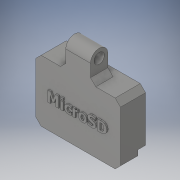
# Autodesk Inventor part: SDCardCover
Saved by Autodesk Inventor 2018 (Build 220112000, 112)
## iProperties
Created: 2019-01-13
Part Number: SDCardCover
Material: Generic
Document SubType Name: Modeling
Designer: tbrow
Density: 1 g/cm^3
Appearance: Default
Author: tbrow
## iProperties of the stored document SDCardCover_3DPrint.ipt
Created: 2019-01-15
Part Number: SDCardCover_3DPrint
Material: Generic
Document SubType Name: Modeling
Designer: tbrow
Density: 1 g/cm^3
Appearance: Default
Author: tbrow
Autodesk Inventor part; units mm, degrees
note: some values were not read from the file. Chosen so that the rebuilt part matches the saved one: direction of "Emboss1".
ref_plane "YZ Plane" through (0, 0, 0) normal (1, 0, 0) x (0, 1, 0)
ref_plane "XZ Plane" through (0, 0, 0) normal (0, 1, 0) x (-1, 0, 0)
ref_plane "XY Plane" through (0, 0, 0) normal (0, 0, 1) x (1, 0, 0)
sketch "Sketch1" plane through (0, 0, 0) normal (0, 0, 1) x (1, 0, 0)
  line L0 (0, 0) -> (0, 22.1234)
  line L1 (0, 22.1234) -> (10.795, 22.1234)
  line L2 (10.795, 22.1234) -> (10.795, 31.6484)
  line L3 (10.795, 31.6484) -> (19.685, 31.6484)
  line L4 (19.685, 31.6484) -> (19.685, 22.1234)
  line L5 (19.685, 22.1234) -> (30.48, 22.1234)
  line L6 (30.48, 22.1234) -> (30.48, 0)
  line L7 (30.48, 0) -> (0, 0)
  dimension "d0" = 10.795
  dimension "d1" = 9.525
  dimension "d2" = 8.89
  dimension "d3" = 10.795
  dimension "d17" = 31.6484
  constraints: 16 end point, 6 perpendicular, 2 point on line, 1 vertical
  measures "d0" distance of L4.end L5.end
  measures "d1" distance of L3.end L4.end
  measures "d2" distance of L2.end L3.end
  measures "d3" distance of L0.end L1.end
  measures "d17" distance between parallel lines of L7 L3
extrude "Extrusion1" add sketch "Sketch1" along normal blind 6.2484
sketch "Sketch2" plane through (19.685, 22.1234, 0) normal (1, 0, 0) x (0, 0, -1)
  circle A0 centre (-3.1242, 6.4008) radius 1.8542
  line L0 (0, 9.525) -> (-6.2484, 9.525) projected
  line L1 (-3.1242, 9.525) -> (-3.1242, 0) construction
  line L2 (0, 0) -> (-6.2484, 0) projected
  point P0 (0, -22.1234)
  dimension "d7" = 3.7084
  dimension "d8" = 3.1242
  constraints: 2 end point, 2 midpoint, 1 centre point, 1 point on line
  measures "d7" diameter of A0
  measures "d8" distance from line of L0 A0.centre
extrude "Extrusion2" cut sketch "Sketch2" against normal through all
fillet "Fillet1" radius 3.1242 2 edges at (15.24, 31.6484, 6.2484) (15.24, 31.6484, 0)
chamfer "Chamfer1" distance 1.905 angle 45 6 edges at (19.685, 22.1234, 3.1242) (10.795, 22.1234, 3.1242) (30.48, 22.1234, 3.1242) (0, 22.1234, 3.1242) (30.48, 0, 3.1242) (0, 0, 3.1242)
sketch "Sketch3" plane through (0, 0, 6.2484) normal (0, 0, 1) x (1, 0, 0)
  line L0 (4.3912, 13.1811) -> (26.0888, 13.1811) construction
  line L1 (26.0888, 13.1811) -> (26.0888, 8.9423) construction
  line L2 (26.0888, 8.9423) -> (4.3912, 8.9423) construction
  line L3 (4.3912, 8.9423) -> (4.3912, 13.1811) construction
  line L4 (4.3912, 11.0617) -> (26.0888, 11.0617) construction
  line L5 (15.24, 13.1811) -> (15.24, 8.9423) construction
  line L6 (19.685, 31.6484) -> (10.795, 31.6484) projected
  line L7 (15.24, 31.6484) -> (15.24, 0) construction
  line L8 (28.575, 0) -> (0, 0) projected
  line L9 (0, 0) -> (0, 20.2184) projected
  line L10 (0, 11.0617) -> (30.48, 11.0617) construction
  line L11 (30.48, 20.2184) -> (30.48, 1.905) projected
  line L12 (8.6766, 9.1982) -> (7.7257, 9.1982)
  line L13 (7.7257, 9.1982) -> (7.7257, 11.7238)
  line L14 (7.7257, 11.7238) -> (7.0341, 10.0936)
  line L15 (7.0341, 10.0936) -> (6.3795, 10.0936)
  line L16 (6.3795, 10.0936) -> (5.6879, 11.7238)
  line L17 (5.6879, 11.7238) -> (5.6879, 9.1982)
  line L18 (5.6879, 9.1982) -> (4.7864, 9.1982)
  line L19 (4.7864, 9.1982) -> (4.7864, 13.0082)
  line L20 (4.7864, 13.0082) -> (5.8886, 13.0082)
  line L21 (5.8886, 13.0082) -> (6.7346, 11.1279)
  line L22 (6.7346, 11.1279) -> (7.5744, 13.0082)
  line L23 (7.5744, 13.0082) -> (8.6766, 13.0082)
  line L24 (8.6766, 13.0082) -> (8.6766, 9.1982)
  line L25 (10.3099, 9.1982) -> (9.4146, 9.1982)
  line L26 (9.4146, 9.1982) -> (9.4146, 12.0727)
  line L27 (9.4146, 12.0727) -> (10.3099, 12.0727)
  line L28 (10.3099, 12.0727) -> (10.3099, 9.1982)
  line L29 (10.3377, 12.4833) -> (9.3899, 12.4833)
  line L30 (9.3899, 12.4833) -> (9.3899, 13.1811)
  line L31 (9.3899, 13.1811) -> (10.3377, 13.1811)
  line L32 (10.3377, 13.1811) -> (10.3377, 12.4833)
  spline S0 degree 2 poles (12.4033, 9.121) (12.0482, 9.121) (11.4585, 9.3001) (11.2393, 9.4853) knots 0 0 0 1 2 2 2
  spline S1 degree 2 poles (11.2393, 9.4853) (11.0262, 9.6737) (10.7854, 10.2387) (10.7854, 10.6216) knots 0 0 0 1 2 2 2
  spline S2 degree 2 poles (10.7854, 10.6216) (10.7854, 11.0353) (11.0448, 11.6126) (11.2702, 11.7979) knots 0 0 0 1 2 2 2
  spline S3 degree 2 poles (11.2702, 11.7979) (11.4832, 11.977) (12.0636, 12.1499) (12.3786, 12.1499) knots 0 0 0 1 2 2 2
  spline S4 degree 2 poles (12.3786, 12.1499) (12.6163, 12.1499) (13.0918, 12.0387) (13.3326, 11.9183) knots 0 0 0 1 2 2 2
  line L33 (13.3326, 11.9183) -> (13.3326, 11.1526)
  line L34 (13.3326, 11.1526) -> (13.2184, 11.1526)
  spline S5 degree 2 poles (13.2184, 11.1526) (13.1628, 11.2051) (13.0084, 11.3286) (12.9158, 11.378) knots 0 0 0 1 2 2 2
  spline S6 degree 2 poles (12.9158, 11.378) (12.817, 11.4336) (12.5731, 11.5077) (12.4218, 11.5077) knots 0 0 0 1 2 2 2
  spline S7 degree 2 poles (12.4218, 11.5077) (12.0791, 11.5077) (11.7024, 11.0291) (11.7024, 10.6216) knots 0 0 0 1 2 2 2
  spline S8 degree 2 poles (11.7024, 10.6216) (11.7024, 10.1893) (12.1038, 9.7632) (12.4372, 9.7632) knots 0 0 0 1 2 2 2
  spline S9 degree 2 poles (12.4372, 9.7632) (12.6071, 9.7632) (12.8602, 9.8404) (12.9529, 9.896) knots 0 0 0 1 2 2 2
  spline S10 degree 2 poles (12.9529, 9.896) (13.0424, 9.9485) (13.1721, 10.0658) (13.2184, 10.1121) knots 0 0 0 1 2 2 2
  line L35 (13.2184, 10.1121) -> (13.3326, 10.1121)
  line L36 (13.3326, 10.1121) -> (13.3326, 9.3433)
  spline S11 degree 2 poles (13.3326, 9.3433) (13.2554, 9.3094) (13.0547, 9.2229) (12.9498, 9.1951) knots 0 0 0 1 2 2 2
  spline S12 degree 2 poles (12.9498, 9.1951) (12.8201, 9.1581) (12.5916, 9.121) (12.4033, 9.121) knots 0 0 0 1 2 2 2
  line L37 (15.6884, 11.2236) -> (15.6143, 11.2236)
  spline S13 degree 2 poles (15.6143, 11.2236) (15.5618, 11.2421) (15.3673, 11.2607) (15.25, 11.2607) knots 0 0 0 1 2 2 2
  spline S14 degree 2 poles (15.25, 11.2607) (15.111, 11.2607) (14.7992, 11.1773) (14.6541, 11.1217) knots 0 0 0 1 2 2 2
  line L38 (14.6541, 11.1217) -> (14.6541, 9.1982)
  line L39 (14.6541, 9.1982) -> (13.7587, 9.1982)
  line L40 (13.7587, 9.1982) -> (13.7587, 12.0727)
  line L41 (13.7587, 12.0727) -> (14.6541, 12.0727)
  line L42 (14.6541, 12.0727) -> (14.6541, 11.659)
  spline S15 degree 2 poles (14.6541, 11.659) (14.7158, 11.7145) (14.932, 11.8874) (15.0215, 11.9399) knots 0 0 0 1 2 2 2
  spline S16 degree 2 poles (15.0215, 11.9399) (15.1203, 11.9986) (15.3796, 12.0819) (15.4939, 12.0819) knots 0 0 0 1 2 2 2
  spline S17 degree 2 poles (15.4939, 12.0819) (15.5371, 12.0819) (15.6452, 12.0758) (15.6884, 12.0727) knots 0 0 0 1 2 2 2
  line L43 (15.6884, 12.0727) -> (15.6884, 11.2236)
  spline S18 degree 2 poles (18.7883, 10.6339) (18.7883, 9.9238) (18.0133, 9.1087) (17.3063, 9.1087) knots 0 0 0 1 2 2 2
  spline S19 degree 2 poles (17.3063, 9.1087) (16.6023, 9.1087) (15.8212, 9.9238) (15.8212, 10.6339) knots 0 0 0 1 2 2 2
  spline S20 degree 2 poles (15.8212, 10.6339) (15.8212, 11.3502) (16.6023, 12.1622) (17.3063, 12.1622) knots 0 0 0 1 2 2 2
  spline S21 degree 2 poles (17.3063, 12.1622) (18.0102, 12.1622) (18.7883, 11.3471) (18.7883, 10.6339) knots 0 0 0 1 2 2 2
  spline S22 degree 2 poles (17.8713, 10.6277) (17.8713, 10.884) (17.7879, 11.2267) (17.7138, 11.3286) knots 0 0 0 1 2 2 2
  spline S23 degree 2 poles (17.7138, 11.3286) (17.6335, 11.4367) (17.4328, 11.52) (17.3063, 11.52) knots 0 0 0 1 2 2 2
  spline S24 degree 2 poles (17.3063, 11.52) (17.1828, 11.52) (16.9882, 11.4459) (16.908, 11.3409) knots 0 0 0 1 2 2 2
  spline S25 degree 2 poles (16.908, 11.3409) (16.8308, 11.2421) (16.7382, 10.8933) (16.7382, 10.6277) knots 0 0 0 1 2 2 2
  spline S26 degree 2 poles (16.7382, 10.6277) (16.7382, 10.3653) (16.8246, 10.0411) (16.8956, 9.9423) knots 0 0 0 1 2 2 2
  spline S27 degree 2 poles (16.8956, 9.9423) (16.9666, 9.8435) (17.1828, 9.7509) (17.3124, 9.7509) knots 0 0 0 1 2 2 2
  spline S28 degree 2 poles (17.3124, 9.7509) (17.4205, 9.7509) (17.6428, 9.8435) (17.7107, 9.9361) knots 0 0 0 1 2 2 2
  spline S29 degree 2 poles (17.7107, 9.9361) (17.7879, 10.0442) (17.8713, 10.356) (17.8713, 10.6277) knots 0 0 0 1 2 2 2
  spline S30 degree 2 poles (20.4926, 9.1303) (20.0542, 9.1303) (19.3934, 9.3001) (19.1094, 9.4236) knots 0 0 0 1 2 2 2
  line L44 (19.1094, 9.4236) -> (19.1094, 10.3313)
  line L45 (19.1094, 10.3313) -> (19.1958, 10.3313)
  spline S31 degree 2 poles (19.1958, 10.3313) (19.483, 10.0874) (20.1715, 9.825) (20.4957, 9.825) knots 0 0 0 1 2 2 2
  spline S32 degree 2 poles (20.4957, 9.825) (20.579, 9.825) (20.8476, 9.862) (20.9279, 9.8991) knots 0 0 0 1 2 2 2
  spline S33 degree 2 poles (20.9279, 9.8991) (21.0267, 9.9423) (21.1657, 10.0998) (21.1657, 10.2263) knots 0 0 0 1 2 2 2
  spline S34 degree 2 poles (21.1657, 10.2263) (21.1657, 10.3715) (20.9403, 10.5505) (20.7859, 10.5907) knots 0 0 0 1 2 2 2
  spline S35 degree 2 poles (20.7859, 10.5907) (20.5914, 10.6432) (20.1499, 10.7327) (19.9554, 10.8006) knots 0 0 0 1 2 2 2
  spline S36 degree 2 poles (19.9554, 10.8006) (19.5138, 10.955) (19.131, 11.483) (19.131, 11.8782) knots 0 0 0 1 2 2 2
  spline S37 degree 2 poles (19.131, 11.8782) (19.131, 12.4123) (20.0356, 13.0761) (20.7149, 13.0761) knots 0 0 0 1 2 2 2
  spline S38 degree 2 poles (20.7149, 13.0761) (21.0545, 13.0761) (21.7276, 12.9372) (21.9931, 12.8199) knots 0 0 0 1 2 2 2
  line L46 (21.9931, 12.8199) -> (21.9931, 11.9492)
  line L47 (21.9931, 11.9492) -> (21.9098, 11.9492)
  spline S39 degree 2 poles (21.9098, 11.9492) (21.6967, 12.1313) (21.0854, 12.3814) (20.7643, 12.3814) knots 0 0 0 1 2 2 2
  spline S40 degree 2 poles (20.7643, 12.3814) (20.6377, 12.3814) (20.4401, 12.3444) (20.3289, 12.295) knots 0 0 0 1 2 2 2
  spline S41 degree 2 poles (20.3289, 12.295) (20.2394, 12.2548) (20.1097, 12.0943) (20.1097, 11.9955) knots 0 0 0 1 2 2 2
  spline S42 degree 2 poles (20.1097, 11.9955) (20.1097, 11.8473) (20.3166, 11.6775) (20.613, 11.6096) knots 0 0 0 1 2 2 2
  spline S43 degree 2 poles (20.613, 11.6096) (20.8044, 11.5663) (21.1595, 11.483) (21.3633, 11.412) knots 0 0 0 1 2 2 2
  spline S44 degree 2 poles (21.3633, 11.412) (21.7585, 11.2668) (22.1444, 10.7852) (22.1444, 10.39) knots 0 0 0 1 2 2 2
  spline S45 degree 2 poles (22.1444, 10.39) (22.1444, 9.8219) (21.2521, 9.1303) (20.4926, 9.1303) knots 0 0 0 1 2 2 2
  spline S46 degree 2 poles (26.0347, 11.1001) (26.0347, 10.566) (25.5685, 9.7262) (25.2134, 9.5008) knots 0 0 0 1 2 2 2
  spline S47 degree 2 poles (25.2134, 9.5008) (24.917, 9.3094) (24.2192, 9.1982) (23.8271, 9.1982) knots 0 0 0 1 2 2 2
  line L48 (23.8271, 9.1982) -> (22.6353, 9.1982)
  line L49 (22.6353, 9.1982) -> (22.6353, 13.0082)
  line L50 (22.6353, 13.0082) -> (23.8148, 13.0082)
  spline S48 degree 2 poles (23.8148, 13.0082) (24.2161, 13.0082) (24.917, 12.9063) (25.2257, 12.7087) knots 0 0 0 1 2 2 2
  spline S49 degree 2 poles (25.2257, 12.7087) (25.5993, 12.4679) (26.0347, 11.6528) (26.0347, 11.1001) knots 0 0 0 1 2 2 2
  spline S50 degree 2 poles (25.0528, 11.1063) (25.0528, 11.483) (24.7935, 12.0202) (24.528, 12.1715) knots 0 0 0 1 2 2 2
  spline S51 degree 2 poles (24.528, 12.1715) (24.3335, 12.2765) (23.9074, 12.2981) (23.611, 12.2981) knots 0 0 0 1 2 2 2
  line L51 (23.611, 12.2981) -> (23.5925, 12.2981)
  line L52 (23.5925, 12.2981) -> (23.5925, 9.9114)
  line L53 (23.5925, 9.9114) -> (23.611, 9.9114)
  spline S52 degree 2 poles (23.611, 9.9114) (23.9321, 9.9114) (24.3736, 9.933) (24.5743, 10.0596) knots 0 0 0 1 2 2 2
  spline S53 degree 2 poles (24.5743, 10.0596) (24.8089, 10.2078) (25.0528, 10.7296) (25.0528, 11.1063) knots 0 0 0 1 2 2 2
  point P0 (30.48, 0)
  point P1 (0, 22.1234)
  point P2 (30.48, 22.1234)
  constraints: 8 end point, 6 midpoint, 2 collinear, 2 point on line, 2 other
emboss "Emboss1" sketch "Sketch3" operation add depth 0.508 direction (0, 0, -1)
sketch "Sketch4" plane through (0, 0, 0) normal (0, 0, -1) x (-1, 0, 0)
  line L0 (-21.59, 22.1234) -> (-8.89, 22.1234)
  line L1 (-1.905, 22.1234) -> (-8.89, 22.1234) projected
  line L2 (-1.905, 22.1234) -> (0, 20.2184) projected
  line L3 (0, 1.905) -> (0, 20.2184) projected
  line L4 (0, 1.905) -> (-1.905, 0) projected
  line L5 (-28.575, 0) -> (-1.905, 0) projected
  line L6 (-28.575, 0) -> (-30.48, 1.905) projected
  line L7 (-30.48, 20.2184) -> (-30.48, 1.905) projected
  line L8 (-30.48, 20.2184) -> (-28.575, 22.1234) projected
  line L9 (-21.59, 22.1234) -> (-28.575, 22.1234) projected
  line L10 (-28.0489, 20.8534) -> (-29.21, 19.6923)
  line L11 (-29.21, 19.6923) -> (-29.21, 2.4311)
  line L12 (-29.21, 2.4311) -> (-28.0489, 1.27)
  line L13 (-28.0489, 1.27) -> (-2.4311, 1.27)
  line L14 (-2.4311, 1.27) -> (-1.27, 2.4311)
  line L15 (-1.27, 2.4311) -> (-1.27, 19.6923)
  line L16 (-1.27, 19.6923) -> (-2.4311, 20.8534)
  line L17 (-2.4311, 20.8534) -> (-8.89, 20.8534)
  line L18 (-8.89, 20.8534) -> (-21.59, 20.8534)
  line L19 (-21.59, 20.8534) -> (-28.0489, 20.8534)
  line L20 (-29.21, 3.175) -> (-1.27, 3.175)
  line L21 (-29.21, 3.81) -> (-30.48, 3.81)
  line L22 (-1.27, 3.81) -> (0, 3.81)
  point P0 (0, 0)
  dimension "d18" = 1.27
  dimension "d19" = 3.175
  dimension "d20" = 0.635
  dimension "d21" = 0.635
  constraints: 28 end point, 6 point on line, 3 perpendicular, 1 horizontal, 9 other
  measures "d18" distance between parallel lines of L9 L19
  measures "d19" distance between parallel lines of L20 L5
  measures "d20" distance between parallel lines of L20 L21
  measures "d21" distance between parallel lines of L22 L20
extrude "Extrusion3" add sketch "Sketch4" along normal blind 2.794 contours L0 L1 L2 L3 L22 L15 L16 L17 L18 L19 L10 L11 L21 L7 L8 L9
body "Solid1"
